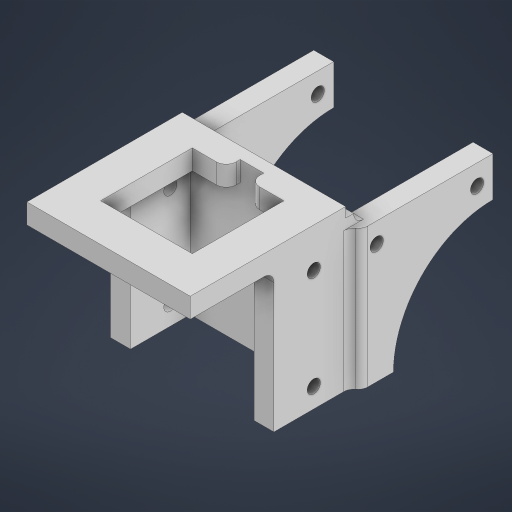
# Autodesk Inventor part: Outer_Tube_Worm_Connector
Saved by Autodesk Inventor 2023 (Build 270158000, 158)
## iProperties
Created: 2024-02-19
Part Number: Outer_Tube_Worm_Connector
Material: Generic
Document SubType Name: Modeling
Designer: kelle
Density: 1 g/cm^3
Appearance: Default
Author: kelle
Autodesk Inventor part; units mm, degrees
ref_plane "YZ Plane" through (0, 0, 0) normal (1, 0, 0) x (0, 1, 0)
ref_plane "XZ Plane" through (0, 0, 0) normal (0, 1, 0) x (-1, 0, 0)
ref_plane "XY Plane" through (0, 0, 0) normal (0, 0, 1) x (1, 0, 0)
sketch "Sketch1" plane through (0, 0, 0) normal (0, 0, 1) x (1, 0, 0)
  line L0 (19.685, -22.225) -> (-19.685, -22.225)
  line L1 (-19.685, -22.225) -> (-19.685, 22.225)
  line L2 (-19.685, 22.225) -> (19.685, 22.225)
  line L3 (19.685, 22.225) -> (19.685, -22.225)
  line L4 (19.685, -22.225) -> (-19.685, 22.225) construction
  line L5 (-19.685, -22.225) -> (19.685, 22.225) construction
  line L6 (-19.685, 22.225) -> (-26.035, 22.225)
  line L7 (-26.035, 22.225) -> (-26.035, -22.225)
  line L8 (-26.035, -22.225) -> (-19.685, -22.225)
  line L9 (-19.685, -22.225) -> (-19.685, 22.225)
  line L10 (19.685, 22.225) -> (26.035, 22.225)
  line L11 (26.035, 22.225) -> (26.035, -22.225)
  line L12 (26.035, -22.225) -> (19.685, -22.225)
  line L13 (19.685, -22.225) -> (19.685, 22.225)
  point P0 (0, 0)
  point P1 (-22.86, -22.225)
  point P2 (19.685, -22.225)
  point P3 (-19.685, -22.225)
  dimension "d0" = 39.37
  dimension "d1" = 44.45
  dimension "d2" = 6.35
  dimension "d3" = 6.35
  dimension "d4" = 44.45
  dimension "d5" = 44.45
  constraints: 28 end point, 6 parallel, 3 horizontal, 3 midpoint, 3 perpendicular
  measures "d0" distance of L1.end L2.end
  measures "d1" distance of L0.end L1.end
  measures "d2" distance of L8.end L7.end
  measures "d3" distance of L11.end L12.end
  measures "d4" distance of L10.end L11.end
  measures "d5" distance from line of L6 point (-22.86, -22.225)
extrude "Extrusion1" add sketch "Sketch1" along normal blind 25.4 contours L3 L10 L11 L12 | L8 L7 L6 L1
extrude "Extrusion2" add sketch "Sketch1" along normal blind 6.35 contours L0 L1 L2 L3
sketch "Sketch2" plane through (26.035, -22.225, 0) normal (1, 0, 0) x (0, 0, -1)
  line L0 (0, 0) -> (0, 44.45) projected
  line L1 (0, 44.45) -> (-25.4, 44.45) projected
  line L2 (-25.4, 0) -> (-25.4, 44.45) projected
  line L3 (0, 0) -> (-25.4, 0) projected
  line L4 (-12.7, 44.45) -> (-12.7, 0) construction
  line L5 (0, 0) -> (-25.4, 0) construction
  line L6 (-25.4, 44.45) -> (-25.4, 0) construction
  line L7 (-25.4, 22.225) -> (0, 22.225) construction
  circle A0 centre (-12.7, 38.227) radius 2.0955
  circle A1 centre (-12.7, 6.223) radius 2.0955
  dimension "d10" = 4.191
  dimension "d11" = 4.191
  dimension "d12" = 32.004
  dimension "d13" = 16.002
  constraints: 4 end point, 3 midpoint, 2 centre point, 2 point on line, 1 horizontal
  measures "d10" diameter of A0
  measures "d11" diameter of A1
  measures "d12" distance of A1.centre A0.centre
  measures "d13" distance from line of L7 A1.centre
extrude "Extrusion3" cut sketch "Sketch2" against normal through all contours A0 | A1
sketch "Sketch6" plane through (0, 0, 0) normal (0, 0, -1) x (-1, 0, 0)
  line L0 (-26.035, 22.225) -> (26.035, 22.225) construction
  line L1 (0, 22.225) -> (0, -22.225) construction
  line L2 (19.685, -22.225) -> (-19.685, -22.225) construction
  line L3 (-26.035, -22.225) -> (-26.035, 22.225) construction
  line L4 (-26.035, 0) -> (26.3172, 0) construction
  line L5 (-22.225, 22.225) -> (-28.575, 22.225)
  line L6 (-28.575, 22.225) -> (-28.575, -22.225)
  line L7 (-28.575, -22.225) -> (-22.225, -22.225)
  line L8 (-22.225, -22.225) -> (-22.225, 22.225)
  line L9 (28.575, 22.225) -> (22.225, 22.225)
  line L10 (22.225, 22.225) -> (22.225, -22.225)
  line L11 (22.225, -22.225) -> (28.575, -22.225)
  line L12 (28.575, -22.225) -> (28.575, 22.225)
  point P0 (0, 0)
  dimension "d36" = 6.35
  dimension "d37" = 6.35
  dimension "d38" = 22.225
  dimension "d39" = 22.225
  constraints: 20 end point, 4 parallel, 3 horizontal, 3 midpoint, 2 perpendicular
  measures "d36" distance of L7.end L6.end
  measures "d37" distance of L11.end L10.end
  measures "d38" distance between parallel lines of L1 L10
  measures "d39" distance between parallel lines of L1 L8
extrude "Extrusion7" add sketch "Sketch6" along normal blind 41.91
sketch "Sketch7" plane through (28.575, -22.225, 0) normal (1, 0, 0) x (0, 0, -1)
  circle A0 centre (4.826, 38.0433) radius 2.0955
  line L0 (-20.2466, 38.0433) -> (41.91, 38.0433) construction
  line L1 (41.91, 0) -> (41.91, 44.45) construction
  circle A1 centre (36.83, 38.0433) radius 2.0955
  point P0 (0, 22.225)
  dimension "d42" = 4.191
  dimension "d43" = 4.191
  dimension "d44" = 32.004
  dimension "d45" = 5.08
  constraints: 2 centre point, 2 end point, 2 point on line, 1 horizontal
  measures "d42" diameter of A0
  measures "d43" diameter of A1
  measures "d44" distance of A0.centre A1.centre
  measures "d45" distance from line of L1 A1.centre
extrude "Extrusion8" cut sketch "Sketch7" against normal through all
sketch "Sketch8" plane through (28.575, -22.225, 0) normal (1, 0, 0) x (0, 0, -1)
  line L0 (41.91, 44.45) -> (41.91, 0) projected
  circle A0 centre (41.91, 0) radius 31.75
  point P0 (0, 22.225)
  dimension "d48" = 63.5
  constraints: 1 centre point
  measures "d48" diameter of A0
extrude "Extrusion9" cut sketch "Sketch8" against normal through all
fillet "Fillet1" radius 3.175 2 edges at (26.035, 0, 0) (28.575, 0, 0)
fillet "Fillet2" radius 3.175 2 edges at (-26.035, 0, 0) (-28.575, 0, 0)
sketch "Sketch9" plane through (-26.035, 22.225, 25.4) normal (0, 1, 0) x (1, 0, 0)
  arc A0 (-2.54, 27.3691) -> (-1.27, 24.8291) centre (0.635, 27.3691) ccw projected
  arc A1 (0, 22.2891) -> (-1.27, 24.8291) centre (-3.175, 22.2891) ccw projected
  line L0 (0, 22.2891) -> (0, 0) projected
  line L1 (6.35, 0) -> (0, 0) projected
  line L2 (6.35, 19.05) -> (6.35, 0) projected
  line L3 (45.72, 19.05) -> (6.35, 19.05) construction
  line L4 (45.72, 19.05) -> (45.72, 0) projected
  line L5 (52.07, 0) -> (45.72, 0) projected
  line L6 (52.07, 22.2891) -> (52.07, 0) projected
  arc A2 (53.34, 24.8291) -> (52.07, 22.2891) centre (55.245, 22.2891) ccw projected
  arc A3 (53.34, 24.8291) -> (54.61, 27.3691) centre (51.435, 27.3691) ccw projected
  line L7 (54.61, 27.3691) -> (54.61, 67.31) projected
  line L8 (48.26, 67.31) -> (54.61, 67.31) projected
  line L9 (48.26, 25.4) -> (48.26, 67.31) projected
  line L10 (48.26, 25.4) -> (3.81, 25.4) projected
  line L11 (3.81, 25.4) -> (3.81, 67.31) projected
  line L12 (-2.54, 67.31) -> (3.81, 67.31) projected
  line L13 (-2.54, 27.3691) -> (-2.54, 67.31) projected
  line L14 (0, 25.4) -> (52.07, 25.4)
  line L15 (52.07, 25.4) -> (52.07, 0)
  line L16 (52.07, 0) -> (0, 0)
  line L17 (0, 0) -> (0, 25.4)
  line L18 (0, 25.4) -> (52.07, 25.4)
  line L19 (52.07, 25.4) -> (52.07, -26.67)
  line L20 (52.07, -26.67) -> (0, -26.67)
  line L21 (0, -26.67) -> (0, 25.4)
  line L22 (6.35, 19.05) -> (45.72, 19.05) projected
  line L23 (26.035, 25.4) -> (26.035, -26.67) construction
  line L24 (0, 0) -> (52.07, 0) construction
  line L25 (40.64, -14.605) -> (11.43, -14.605)
  line L26 (11.43, -14.605) -> (11.43, 14.605)
  line L27 (11.43, 14.605) -> (40.64, 14.605)
  line L28 (40.64, 14.605) -> (40.64, -14.605)
  line L29 (40.64, -14.605) -> (11.43, 14.605) construction
  line L30 (11.43, -14.605) -> (40.64, 14.605) construction
  line L31 (22.285, 14.605) -> (29.785, 14.605) construction
  line L32 (29.785, 14.605) -> (29.785, 19.05)
  line L33 (29.785, 19.05) -> (22.285, 19.05) construction
  line L34 (22.285, 19.05) -> (22.285, 14.605)
  point P0 (26.035, 0)
  point P1 (29.785, 16.8275)
  dimension "d53" = 52.07
  dimension "d55" = 29.21
  dimension "d56" = 29.21
  dimension "d57" = 7.5
  dimension "d58" = 3.75
  constraints: 40 end point, 8 parallel, 5 midpoint, 4 horizontal, 4 perpendicular, 2 point on line, 1 collinear
  measures "d53" distance of L18.end L19.end
  measures "d55" distance of L26.end L27.end
  measures "d56" distance of L25.end L26.end
  measures "d57" distance of L33.end L32.end
  measures "d58" distance from line of L23 point (29.785, 16.828)
extrude "Extrusion10" add sketch "Sketch9" along normal blind 6.35 contours L17 L14 L10 L15 L6 L5 L4 L22 L2 L1 L0 | L1 L16 L26 L25 L28 L5 L19 L20 L21 | L2 L22 L34 L27 L26 L16 | L28 L27 L32 L22 L4 L16
fillet "Fillet3" radius 3.175 4 edges at (24.13, 22.225, 0) (-24.13, 22.225, 0) (22.86, 22.225, 25.4) (-22.86, 22.225, 25.4)
fillet "Fillet4" radius 3.175 2 edges at (-3.75, 25.4, 10.795) (3.75, 25.4, 10.795)
sketch "Sketch10" plane through (0, 0, 0) normal (0, 0, -1) x (-1, 0, 0)
  line L0 (22.225, -22.225) -> (22.225, 25.4) projected
  line L1 (26.035, 25.4) -> (22.225, 25.4) projected
  line L2 (26.035, 25.4) -> (26.035, 28.575) projected
  line L3 (-26.035, 28.575) -> (26.035, 28.575) projected
  line L4 (-26.035, 25.4) -> (-26.035, 28.575) projected
  line L5 (-22.225, 25.4) -> (-26.035, 25.4) projected
  line L6 (-22.225, 25.4) -> (-22.225, -22.225) projected
  line L7 (22.225, -22.225) -> (-22.225, -22.225) projected
  point P0 (0, 0)
extrude "Extrusion11" cut sketch "Sketch10" against normal blind 2.54
body "Solid1"
